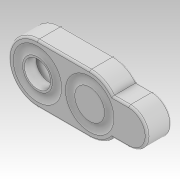
# Autodesk Inventor part: ValveThing
Saved by Autodesk Inventor 2020 (Build 240168000, 168)
## iProperties
Created: 2022-02-05
Part Number: ValveThing
Material: Generic
Document SubType Name: Modeling
Designer: DDeGo
Density: 1 g/cm^3
Appearance: Default
Author: DDeGo
Autodesk Inventor part; units mm, degrees
ref_plane "YZ Plane" through (0, 0, 0) normal (1, 0, 0) x (0, 1, 0)
ref_plane "XZ Plane" through (0, 0, 0) normal (0, 1, 0) x (-1, 0, 0)
ref_plane "XY Plane" through (0, 0, 0) normal (0, 0, 1) x (1, 0, 0)
sketch "Sketch1" plane through (0, 0, 0) normal (0, 0, 1) x (1, 0, 0)
  line L0 (0, 0) -> (4, 0) construction
  line L1 (0, -2.25) -> (4, -2.25)
  line L2 (4, 2.25) -> (0, 2.25)
  arc A0 (0, 2.25) -> (0, -2.25) centre (0, 0) ccw
  arc A1 (4, -2.25) -> (4, 2.25) centre (4, 0) ccw
  line L3 (2, 0) -> (7, 0) construction
  line L4 (2, -1.4) -> (7, -1.4)
  line L5 (7, 1.4) -> (2, 1.4)
  arc A2 (2, 1.4) -> (2, -1.4) centre (2, 0) ccw
  arc A3 (7, -1.4) -> (7, 1.4) centre (7, 0) ccw
  point P0 (4.5, 0)
  point P1 (5.7614, -1.4)
  point P2 (5.7614, 1.4)
  dimension "d0" = 2.25
  dimension "d1" = 1.4
  dimension "d2" = 4
  dimension "d3" = 7
  constraints: 16 end point, 8 point on circle, 8 tangent, 4 centre point, 2 midpoint, 2 parallel, 1 horizontal, 1 point on line
  measures "d0" radius of A0
  measures "d1" radius of A3
  measures "d2" distance of L0.start L0.end
  measures "d3" distance of L3.end L0.start
extrude "Extrusion1" add sketch "Sketch1" along normal blind 1.9
sketch "Sketch2" plane through (0, 0, 1.9) normal (0, 0, 1) x (1, 0, 0)
  circle A0 centre (0, 0) radius 1
  dimension "d6" = 2
  constraints: 1 centre point, 1 coincident
  measures "d6" diameter of A0
extrude "Extrusion2" cut sketch "Sketch2" against normal blind 0.9
sketch "Sketch3" plane through (0, 0, 0) normal (0, 0, -1) x (-1, 0, 0)
  line L0 (-0.4, 0) -> (-3, 0) construction
  line L1 (-0.4, 0.8) -> (-3, 0.8)
  line L2 (-3, -0.8) -> (-0.4, -0.8)
  arc A0 (-0.4, -0.8) -> (-0.4, 0.8) centre (-0.4, 0) ccw
  arc A1 (-3, 0.8) -> (-3, -0.8) centre (-3, 0) ccw
  point P0 (0, 0)
  point P1 (-1.7, 0)
  dimension "d10" = 3
  dimension "d11" = 0.8
  dimension "d18" = 0.4
  constraints: 8 end point, 4 point on circle, 4 tangent, 2 centre point, 1 horizontal, 1 midpoint, 1 parallel, 1 point on line
  measures "d10" distance of point (0, 0) L0.end
  measures "d11" radius of A0
  measures "d18" distance of L0.start point (0, 0)
extrude "Extrusion3" cut sketch "Sketch3" against normal blind 1
fillet "Fillet1" radius 0.6 2 edges at (0.8944, -0.4472, 1) (0.8944, 0.4472, 1)
sketch "Sketch5" plane through (0, 0, 0) normal (0, 0, -1) x (-1, 0, 0)
  line L0 (-5, -0.75) -> (-7.5, -0.75) construction
  line L1 (-5, -0.55) -> (-7.5, -0.55)
  line L2 (-7.5, -0.95) -> (-5, -0.95)
  arc A0 (-5, -0.95) -> (-5, -0.55) centre (-5, -0.75) ccw
  arc A1 (-7.5, -0.55) -> (-7.5, -0.95) centre (-7.5, -0.75) ccw
  line L3 (-5, 0) -> (-7.8, 0) construction
  line L4 (-5, 0.2) -> (-7.8, 0.2)
  line L5 (-7.8, -0.2) -> (-5, -0.2)
  arc A2 (-5, -0.2) -> (-5, 0.2) centre (-5, 0) ccw
  arc A3 (-7.8, 0.2) -> (-7.8, -0.2) centre (-7.8, 0) ccw
  line L6 (-5, 0.75) -> (-7.5, 0.75) construction
  line L7 (-5, 0.95) -> (-7.5, 0.95)
  line L8 (-7.5, 0.55) -> (-5, 0.55)
  arc A4 (-5, 0.55) -> (-5, 0.95) centre (-5, 0.75) ccw
  arc A5 (-7.5, 0.95) -> (-7.5, 0.55) centre (-7.5, 0.75) ccw
  line L9 (-5, 0.75) -> (-5, 0) construction
  line L10 (-5, 0) -> (-5, -0.75) construction
  line L11 (-7.5, -0.75) -> (-7.5, 0.75) construction
  arc A6 (-7, 1.4) -> (-7, -1.4) centre (-7, 0) ccw projected
  line L12 (-0.3, -1.5) -> (-4.5, -1.5) construction
  line L13 (-0.3, -1.7) -> (-4.5, -1.7)
  line L14 (-4.5, -1.3) -> (-0.3, -1.3)
  arc A7 (-0.3, -1.7) -> (-0.3, -1.3) centre (-0.3, -1.5) ccw
  arc A8 (-4.5, -1.3) -> (-4.5, -1.7) centre (-4.5, -1.5) ccw
  line L15 (-0.3, 1.5) -> (-4.5, 1.5) construction
  line L16 (-0.3, 1.3) -> (-4.5, 1.3)
  line L17 (-4.5, 1.7) -> (-0.3, 1.7)
  arc A9 (-0.3, 1.3) -> (-0.3, 1.7) centre (-0.3, 1.5) ccw
  arc A10 (-4.5, 1.7) -> (-4.5, 1.3) centre (-4.5, 1.5) ccw
  line L18 (-4.5, -1.5) -> (-4.5, 1.5) construction
  line L19 (-0.3, 1.5) -> (-0.3, -1.5) construction
  line L20 (-4, 2.25) -> (0, 2.25) projected
  line L21 (0, -2.25) -> (-4, -2.25) projected
  point P0 (0, 0)
  point P1 (-6.25, -0.75)
  point P2 (-6.4, 0)
  point P3 (-6.25, 0.75)
  point P4 (-2.4, -1.5)
  point P5 (-2.4, 1.5)
  dimension "d20" = 0.8
  dimension "d21" = 0.5
  dimension "d22" = 0.75
  dimension "d23" = 0.75
  dimension "d24" = 0.2
  dimension "d25" = 2
  dimension "d37" = 0.3
  dimension "d38" = 0.5
  dimension "d39" = 0.75
  dimension "d40" = 0.75
  constraints: 50 end point, 20 point on circle, 20 tangent, 10 centre point, 8 parallel, 5 midpoint, 4 equal radius, 4 perpendicular, 2 horizontal, 1 point on line, 1 vertical
  measures "d20" distance of L3.end A6.centre
  measures "d21" distance from line of A6.centre L11
  measures "d22" distance between parallel lines of L0 L3
  measures "d23" distance between parallel lines of L6 L3
  measures "d24" radius of A3
  measures "d25" distance from line of A6.centre L9
  measures "d37" distance from line of L19 point (0, 0)
  measures "d38" distance between parallel lines of L9 L18
  measures "d39" distance between parallel lines of L20 L15
  measures "d40" distance between parallel lines of L21 L12
extrude "Extrusion5" cut sketch "Sketch5" against normal blind 0.3
fillet "Fillet2" radius 0.6 3 edges at (0.5, 0.8, 1) (0.5, -0.8, 1) (-0.4, 0, 1)
fillet "Fillet3" radius 0.15 16 edges at (2, 2.25, 0) (-2.25, 0, 0) (2, -2.25, 0) (4.9779, -2.0264, 0) (4.9779, 2.0264, 0) (8.4, 0, 0) (6.3807, -1.4, 0) (6.3807, 1.4, 0) (8.4, 0, 1.9) (6.3807, -1.4, 1.9) (6.3807, 1.4, 1.9) (2, 2.25, 1.9) (-2.25, 0, 1.9) (2, -2.25, 1.9) (4.9779, -2.0264, 1.9) (4.9779, 2.0264, 1.9)
sketch "Sketch6" plane through (0, 0, 0) normal (0, 1, 0) x (-1, 0, 0)
  circle A0 centre (1.5, 2.25) radius 0.5
  line L0 (0, 3.3) -> (0, -0.55) construction
  line L1 (0, 1.9) -> (2.1, 1.9) construction
  line L2 (1.7582, 1.75) -> (1.1081, 1.75) construction
  point P0 (0, 0)
  dimension "d30" = 1
  dimension "d31" = 1.5
  dimension "d32" = 0.15
  constraints: 2 end point, 1 centre point, 1 horizontal, 1 tangent
  measures "d30" diameter of A0
  measures "d31" distance from line of L0 A0.centre
  measures "d32" distance between parallel lines of L1 L2
revolve "Revolution1" cut sketch "Sketch6" angle 360 about axis through (0, 0, 1.9) along (0, 0, -1)
pattern_linear "Rectangular Pattern1" count 2 spacing 4 along (1, 0, 0) of "Revolution1"
sketch "Sketch7" plane through (0, -2.25, 1.75) normal (0, -1, 0) x (1, 0, 0)
  line L0 (0.7066, -0.187) -> (6.5507, -0.187) construction
  line L1 (6.5507, -0.187) -> (6.5507, -3.2448) construction
  line L2 (6.5507, -3.2448) -> (0.7066, -3.2448) construction
  line L3 (0.7066, -3.2448) -> (0.7066, -0.187) construction
  line L4 (1.4983, -1.2072) -> (0.8379, -1.2072)
  line L5 (0.8379, -1.2072) -> (0.8379, -1.033)
  line L6 (0.8379, -1.033) -> (1.0486, -1.033)
  line L7 (1.0486, -1.033) -> (1.0486, -0.5038)
  line L8 (1.0486, -0.5038) -> (0.8379, -0.5038)
  line L9 (0.8379, -0.5038) -> (0.8379, -0.3409)
  spline S0 degree 2 poles (0.8379, -0.3409) (0.8841, -0.3409) (0.9756, -0.3288) (1.0032, -0.3158) knots 0 0 0 1 2 2 2
  spline S1 degree 2 poles (1.0032, -0.3158) (1.0348, -0.2996) (1.0705, -0.2453) (1.0737, -0.2048) knots 0 0 0 1 2 2 2
  line L10 (1.0737, -0.2048) -> (1.2925, -0.2048)
  line L11 (1.2925, -0.2048) -> (1.2925, -1.033)
  line L12 (1.2925, -1.033) -> (1.4983, -1.033)
  line L13 (1.4983, -1.033) -> (1.4983, -1.2072)
  line L14 (1.9157, -1.2072) -> (1.6782, -1.2072)
  line L15 (1.6782, -1.2072) -> (1.6782, -0.943)
  line L16 (1.6782, -0.943) -> (1.9157, -0.943)
  line L17 (1.9157, -0.943) -> (1.9157, -1.2072)
  spline S2 degree 2 poles (2.8225, -0.6513) (2.8225, -0.7785) (2.7633, -0.9908) (2.7009, -1.067) knots 0 0 0 1 2 2 2
  spline S3 degree 2 poles (2.7009, -1.067) (2.6361, -1.144) (2.4448, -1.2267) (2.3055, -1.2267) knots 0 0 0 1 2 2 2
  spline S4 degree 2 poles (2.3055, -1.2267) (2.2585, -1.2267) (2.1564, -1.2145) (2.1393, -1.2096) knots 0 0 0 1 2 2 2
  line L18 (2.1393, -1.2096) -> (2.1393, -1.0135)
  line L19 (2.1393, -1.0135) -> (2.1588, -1.0135)
  spline S5 degree 2 poles (2.1588, -1.0135) (2.1774, -1.0233) (2.2471, -1.0443) (2.3079, -1.0443) knots 0 0 0 1 2 2 2
  spline S6 degree 2 poles (2.3079, -1.0443) (2.3573, -1.0443) (2.4489, -1.0184) (2.4813, -0.99) knots 0 0 0 1 2 2 2
  spline S7 degree 2 poles (2.4813, -0.99) (2.5162, -0.9601) (2.5615, -0.8717) (2.5696, -0.8053) knots 0 0 0 1 2 2 2
  spline S8 degree 2 poles (2.5696, -0.8053) (2.5162, -0.8385) (2.4238, -0.8742) (2.3549, -0.8742) knots 0 0 0 1 2 2 2
  spline S9 degree 2 poles (2.3549, -0.8742) (2.3038, -0.8742) (2.209, -0.8466) (2.1701, -0.8174) knots 0 0 0 1 2 2 2
  spline S10 degree 2 poles (2.1701, -0.8174) (2.1183, -0.7777) (2.0575, -0.6505) (2.0575, -0.55) knots 0 0 0 1 2 2 2
  spline S11 degree 2 poles (2.0575, -0.55) (2.0575, -0.4714) (2.111, -0.3393) (2.1596, -0.2907) knots 0 0 0 1 2 2 2
  spline S12 degree 2 poles (2.1596, -0.2907) (2.2082, -0.2421) (2.3492, -0.187) (2.4359, -0.187) knots 0 0 0 1 2 2 2
  spline S13 degree 2 poles (2.4359, -0.187) (2.5235, -0.187) (2.6588, -0.2356) (2.7074, -0.2866) knots 0 0 0 1 2 2 2
  spline S14 degree 2 poles (2.7074, -0.2866) (2.7641, -0.3434) (2.8225, -0.5233) (2.8225, -0.6513) knots 0 0 0 1 2 2 2
  spline S15 degree 2 poles (2.5737, -0.614) (2.5737, -0.5322) (2.5461, -0.4268) (2.521, -0.3977) knots 0 0 0 1 2 2 2
  spline S16 degree 2 poles (2.521, -0.3977) (2.504, -0.3758) (2.4602, -0.3571) (2.4351, -0.3571) knots 0 0 0 1 2 2 2
  spline S17 degree 2 poles (2.4351, -0.3571) (2.4124, -0.3571) (2.3703, -0.375) (2.3508, -0.3977) knots 0 0 0 1 2 2 2
  spline S18 degree 2 poles (2.3508, -0.3977) (2.3338, -0.4171) (2.3095, -0.4925) (2.3095, -0.537) knots 0 0 0 1 2 2 2
  spline S19 degree 2 poles (2.3095, -0.537) (2.3095, -0.5857) (2.3346, -0.6481) (2.3557, -0.6667) knots 0 0 0 1 2 2 2
  spline S20 degree 2 poles (2.3557, -0.6667) (2.3776, -0.6853) (2.4319, -0.6999) (2.4659, -0.6999) knots 0 0 0 1 2 2 2
  spline S21 degree 2 poles (2.4659, -0.6999) (2.4943, -0.6999) (2.5534, -0.6845) (2.5721, -0.6764) knots 0 0 0 1 2 2 2
  spline S22 degree 2 poles (2.5721, -0.6764) (2.5721, -0.6691) (2.5737, -0.6416) (2.5737, -0.614) knots 0 0 0 1 2 2 2
  point P0 (0, -1.75)
  constraints: 2 other
extrude "Extrusion6" cut sketch "Sketch7" against normal blind 0.2
body "Solid1"
